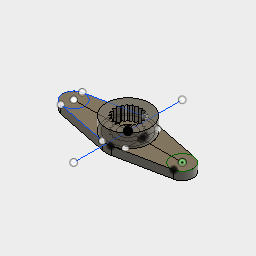
SG-90 (Autodesk Fusion 360 design; units mm, degrees)
Autodesk Fusion 360 part; units mm, degrees
sketch "Sketch1" plane through (0, 0, 0) normal (0, 1, 0) x (1, 0, 0)
  line L0 (2.5, 0.002) -> (2.5, 0.002)
  line L1 (2.5, -2.998) -> (2.5, 3.002)
  line L2 (2.3875, 0.7415) -> (2.1157, 0.3219)
  line L3 (2.1157, 0.3219) -> (2.5, 0.002)
  line L4 (2.0629, 1.4123) -> (1.9268, 0.9312)
  line L5 (1.9268, 0.9312) -> (2.3883, 0.7388)
  line L6 (1.5549, 1.9576) -> (1.5667, 1.4577)
  line L7 (1.5667, 1.4577) -> (2.0645, 1.41)
  line L8 (0.9088, 2.329) -> (1.0675, 1.8548)
  line L9 (1.0675, 1.8548) -> (1.5571, 1.9558)
  line L10 (0.182, 2.4934) -> (0.4733, 2.087)
  line L11 (0.4733, 2.087) -> (0.9115, 2.3279)
  line L12 (-0.561, 2.4362) -> (-0.1629, 2.1338)
  line L13 (-0.1629, 2.1338) -> (0.1848, 2.4932)
  line L14 (-1.2542, 2.1626) -> (-0.7846, 1.991)
  line L15 (-0.7846, 1.991) -> (-0.5583, 2.4369)
  line L16 (-1.8359, 1.6969) -> (-1.3366, 1.6713)
  line L17 (-1.3366, 1.6713) -> (-1.2518, 2.1641)
  line L18 (-2.2545, 1.0803) -> (-1.7698, 1.2031)
  line L19 (-1.7698, 1.2031) -> (-1.834, 1.6989)
  line L20 (-2.4728, 0.3678) -> (-2.0458, 0.628)
  line L21 (-2.0458, 0.628) -> (-2.2533, 1.0829)
  line L22 (-2.4714, -0.3774) -> (-2.14, -0.0029)
  line L23 (-2.14, -0.0029) -> (-2.4724, 0.3706)
  line L24 (-2.2503, -1.0891) -> (-2.0441, -0.6336)
  line L25 (-2.0441, -0.6336) -> (-2.4718, -0.3746)
  line L26 (-1.8293, -1.704) -> (-1.7665, -1.2079)
  line L27 (-1.7665, -1.2079) -> (-2.2515, -1.0865)
  line L28 (-1.2458, -2.1675) -> (-1.332, -1.675)
  line L29 (-1.332, -1.675) -> (-1.8313, -1.7019)
  line L30 (-0.5516, -2.4384) -> (-0.7791, -1.9932)
  line L31 (-0.7791, -1.9932) -> (-1.2482, -2.1661)
  line L32 (0.1917, -2.4926) -> (-0.157, -2.1343)
  line L33 (-0.157, -2.1343) -> (-0.5543, -2.4378)
  line L34 (0.9179, -2.3254) -> (0.4791, -2.0857)
  line L35 (0.4791, -2.0857) -> (0.1888, -2.4929)
  line L36 (1.5625, -1.9516) -> (1.0726, -1.8518)
  line L37 (1.0726, -1.8518) -> (0.9152, -2.3264)
  line L38 (2.0683, -1.4043) -> (1.5707, -1.4534)
  line L39 (1.5707, -1.4534) -> (1.5603, -1.9533)
  line L40 (2.3904, -0.7323) -> (1.9294, -0.9259)
  line L41 (1.9294, -0.9259) -> (2.0667, -1.4066)
  line L42 (2.5, 0.0048) -> (2.1166, -0.316)
  line L43 (2.1166, -0.316) -> (2.3895, -0.7349)
  arc A0 (2.0645, 1.41) -> (2.0629, 1.4123) centre (0, 0) ccw
  arc A1 (1.5571, 1.9558) -> (1.5549, 1.9576) centre (0, 0) ccw
  arc A2 (0.9115, 2.3279) -> (0.9088, 2.329) centre (0, 0) ccw
  arc A3 (0.1848, 2.4932) -> (0.182, 2.4934) centre (0, 0) ccw
  arc A4 (-0.5583, 2.4369) -> (-0.561, 2.4362) centre (0, 0) ccw
  arc A5 (-1.2518, 2.1641) -> (-1.2542, 2.1626) centre (0, 0) ccw
  arc A6 (-1.834, 1.6989) -> (-1.8359, 1.6969) centre (0, 0) ccw
  arc A7 (-2.2533, 1.0829) -> (-2.2545, 1.0803) centre (0, 0) ccw
  arc A8 (-2.4724, 0.3706) -> (-2.4728, 0.3678) centre (0, 0) ccw
  arc A9 (-2.4718, -0.3746) -> (-2.4714, -0.3774) centre (0, 0) ccw
  arc A10 (-2.2515, -1.0865) -> (-2.2503, -1.0891) centre (0, 0) ccw
  arc A11 (-1.8313, -1.7019) -> (-1.8293, -1.704) centre (0, 0) ccw
  arc A12 (-1.2482, -2.1661) -> (-1.2458, -2.1675) centre (0, 0) ccw
  arc A13 (-0.5543, -2.4378) -> (-0.5516, -2.4384) centre (0, 0) ccw
  arc A14 (0.1888, -2.4929) -> (0.1917, -2.4926) centre (0, 0) ccw
  arc A15 (0.9152, -2.3264) -> (0.9179, -2.3254) centre (0, 0) ccw
  arc A16 (1.5603, -1.9533) -> (1.5625, -1.9516) centre (0, 0) ccw
  arc A17 (2.0667, -1.4066) -> (2.0683, -1.4043) centre (0, 0) ccw
  arc A18 (2.3895, -0.7349) -> (2.3904, -0.7323) centre (0, 0) ccw
  arc A19 (2.5, 0) -> (2.5, 0.002) centre (0, 0) ccw
  circle A20 centre (0, 0) radius 4
  circle A21 centre (10, 0) radius 2
  line L44 (10.4, 1.9596) -> (0.8, 3.9192)
  line L45 (-10, 0) -> (10, 0)
  line L46 (0, -10) -> (0, 10)
  line L47 (-10.4, 1.9596) -> (-0.8, 3.9192)
  line L48 (10.4, -1.9596) -> (0.8, -3.9192)
  line L49 (-10.4, -1.9596) -> (-0.8, -3.9192)
  circle A22 centre (-10, 0) radius 2
  circle A23 centre (0, 0) radius 1.5
  circle A24 centre (0, 0) radius 3.5
  point P0 (2.5, 0.002)
  dimension "d1" = 5
  dimension "d3" = 0.748
  dimension "d6" = 0.5
  dimension "d7" = 0.5
  dimension "d9" = 360
  dimension "d10" = 8
  dimension "d11" = 4
  dimension "d12" = 3
  dimension "d13" = 7
  measures "d1" diameter of A0
  measures "d3" distance of P0 L2.start
  measures "d6" distance of L2.start L2.end
  measures "d7" distance of L2.end P0
  measures "d10" diameter of A20
  measures "d11" diameter of A21
  measures "d12" diameter of A23
  measures "d13" diameter of A24
extrude "Extrude1" add sketch "Sketch1" along normal blind 2.5 contours L1 L32 L34 L35 L36 L37 L38 L39 L40 L41 L42 L43 L46 A24 | L1 L45 A24 | L1 L2 L3 L4 L5 L6 L7 L8 L9 L10 L11 L13 L46 A24 | L1 L45 A24 | L22 L23 L24 L25 L26 L27 L28 L29 L30 L31 L32 L33 L45 L46 A24 | L12 L13 L14 L15 L16 L17 L18 L19 L20 L21 L23 L45 L46 A24 makes body 1
extrude "Extrude2" add sketch "Sketch1" along normal blind 2.5 separate body contours A20 L45 L46 A24 | A20 L45 L46 A24 | A20 L45 L46 A24 | A20 L45 L46 A24 makes body 2
extrude "Extrude3" add sketch "Sketch1" against normal blind 1.5 contours L1 L45 A24 | L1 A19 L45 A24 | L1 L32 L34 L35 L36 L37 L38 L39 L40 L41 L42 L43 L45 L46 A24 | A20 L45 L46 A24 | A20 L45 L46 A24 | L2 L3 L4 L5 L6 L7 L8 L9 L10 L11 L13 L42 L45 L46 A23 | L32 L34 L35 L36 L37 L38 L39 L40 L41 L42 L43 L45 L46 A23 | L1 L2 L3 L4 L5 L6 L7 L8 L9 L10 L11 L13 L42 L46 A24 | L22 L23 L24 L25 L26 L27 L28 L29 L30 L31 L32 L33 L45 L46 A24 | A20 L45 L46 A24 | A20 A21 L45 L48 | A20 A21 L44 L45 | L22 L23 L24 L25 L26 L27 L28 L29 L30 L31 L32 L33 L45 L46 A23 | L12 L13 L14 L15 L16 L17 L18 L19 L20 L21 L23 L45 L46 A24 | A20 L45 L46 A24 | A21 | L12 L13 L14 L15 L16 L17 L18 L19 L20 L21 L23 L45 L46 A23 | A20 L45 L49 A22 | A20 L45 L47 A22 | A22 bodies 2 1
extrude "Extrude4" add sketch "Sketch1" along normal blind 0.5 separate body contours L1 L45 A24 | L1 A19 L45 A24 | L1 L32 L34 L35 L36 L37 L38 L39 L40 L41 L42 L43 L45 L46 A24 | L2 L3 L4 L5 L6 L7 L8 L9 L10 L11 L13 L42 L45 L46 A23 | L32 L34 L35 L36 L37 L38 L39 L40 L41 L42 L43 L45 L46 A23 | L1 L2 L3 L4 L5 L6 L7 L8 L9 L10 L11 L13 L42 L46 A24 | L22 L23 L24 L25 L26 L27 L28 L29 L30 L31 L32 L33 L45 L46 A24 | L22 L23 L24 L25 L26 L27 L28 L29 L30 L31 L32 L33 L45 L46 A23 | L12 L13 L14 L15 L16 L17 L18 L19 L20 L21 L23 L45 L46 A24 | L12 L13 L14 L15 L16 L17 L18 L19 L20 L21 L23 L45 L46 A23 makes body 3
move_body "Move1" bodies 3 to x (1, 0, 0) y (0, 1, 0) z (0, 0, 1) at (0, -1.5, 0)
combine "Combine1" operation cut target body 2 tool bodies 3
equation "d3 = ( 5 * PI / 21 ) * 1 mm"
equation "d7 = d6"
